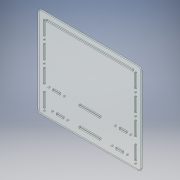
# Autodesk Inventor part: Tapa_Frontal
Saved by Autodesk Inventor 2019 (Build 230136000, 136)
## iProperties
Created: 2020-04-07
Part Number: Tapa_Frontal
Material: Generic
Document SubType Name: Modeling
Designer: Jurgen
Density: 1 g/cm^3
Appearance: Clear
Author: Jurgen
Autodesk Inventor part; units mm, degrees
ref_plane "YZ Plane" through (0, 0, 0) normal (1, 0, 0) x (0, 1, 0)
ref_plane "XZ Plane" through (0, 0, 0) normal (0, 1, 0) x (-1, 0, 0)
ref_plane "XY Plane" through (0, 0, 0) normal (0, 0, 1) x (1, 0, 0)
sketch "Sketch1" plane through (0, 0, 0) normal (0, 0, 1) x (1, 0, 0)
  line L0 (0, 0) -> (20, 0)
  line L1 (0, 0) -> (0, -5)
  line L2 (20, -5) -> (0, -5)
  line L3 (20, 0) -> (20, -5)
  line L4 (76, 0) -> (76, -5)
  line L5 (76, 0) -> (136, 0)
  line L6 (136, -5) -> (76, -5)
  line L7 (136, 0) -> (136, -5)
  line L8 (192, 0) -> (192, -5)
  line L9 (212, 0) -> (192, 0)
  line L10 (212, -5) -> (192, -5)
  line L11 (212, 0) -> (212, -5)
  line L12 (10, -55) -> (10, -60)
  line L13 (30, -55) -> (10, -55)
  line L14 (30, -60) -> (10, -60)
  line L15 (30, -55) -> (30, -60)
  line L16 (76, -55) -> (76, -60)
  line L17 (76, -55) -> (136, -55)
  line L18 (136, -60) -> (76, -60)
  line L19 (136, -55) -> (136, -60)
  line L20 (182, -55) -> (182, -60)
  line L21 (182, -55) -> (202, -55)
  line L22 (202, -60) -> (182, -60)
  line L23 (202, -55) -> (202, -60)
  line L24 (236, -70.0001) -> (236, -80.0001) construction
  line L25 (239.5, -70.0001) -> (236, -70.0001) construction
  line L26 (239.5, -70.0001) -> (239.5, -80.0001) construction
  line L27 (236, -80.0001) -> (239.5, -80.0001) construction
  line L28 (-27.5, -80) -> (-27.5, -70) construction
  line L29 (-24, -70) -> (-27.5, -70) construction
  line L30 (-24, -70) -> (-24, -80) construction
  line L31 (-24, -80) -> (-27.5, -80) construction
  line L32 (-27.5, -60) -> (-27.5, -20)
  line L33 (-24, -20) -> (-27.5, -20)
  line L34 (-24, -60) -> (-24, -20)
  line L35 (-24, -60) -> (-27.5, -60)
  line L36 (-27.5, 0) -> (-27.5, 40)
  line L37 (-24, 40) -> (-24, 0)
  line L38 (-24, 40) -> (-27.5, 40)
  line L39 (-24, 0) -> (-27.5, 0)
  line L40 (-27.5, 60) -> (-27.5, 100)
  line L41 (-24, 100) -> (-27.5, 100)
  line L42 (-24, 100) -> (-24, 60)
  line L43 (-24, 60) -> (-27.5, 60)
  line L44 (-27.5, 160) -> (-27.5, 120)
  line L45 (-24, 160) -> (-24, 120)
  line L46 (-24, 160) -> (-27.5, 160)
  line L47 (236, -0.0001) -> (236, 39.9999)
  line L48 (239.5, 39.9999) -> (239.5, -0.0001)
  line L49 (239.5, 39.9999) -> (236, 39.9999)
  line L50 (239.5, -0.0001) -> (236, -0.0001)
  line L51 (236, -60.0001) -> (236, -20.0001)
  line L52 (239.5, -60.0001) -> (239.5, -20.0001)
  line L53 (239.5, -20.0001) -> (236, -20.0001)
  line L54 (239.5, -60.0001) -> (236, -60.0001)
  line L55 (239.5, 99.9999) -> (236, 99.9999)
  line L56 (236, 59.9999) -> (236, 99.9999)
  line L57 (239.5, 99.9999) -> (239.5, 59.9999)
  line L58 (239.5, 59.9999) -> (236, 59.9999)
  line L59 (236, 159.9999) -> (236, 119.9999)
  line L60 (239.5, 159.9999) -> (239.5, 119.9999)
  line L61 (236, 159.9999) -> (239.5, 159.9999)
  line L62 (236, 111.9999) -> (239.5, 111.9999) construction
  line L63 (239.5, 107.9999) -> (236, 107.9999) construction
  line L64 (236, 51.9999) -> (239.5, 51.9999) construction
  line L65 (239.5, 47.9999) -> (236, 47.9999) construction
  line L66 (236, -66.0001) -> (239.5, -66.0001) construction
  line L67 (212, -60) -> (212, -55) construction
  line L68 (216, -55) -> (216, -60) construction
  line L69 (168, -60) -> (168, -55) construction
  line L70 (172, -55) -> (172, -60) construction
  line L71 (40, -60) -> (40, -55) construction
  line L72 (44, -55) -> (44, -60) construction
  line L73 (-4, -60) -> (-4, -55) construction
  line L74 (0, -55) -> (0, -60) construction
  line L75 (-14, -5) -> (-14, 0) construction
  line L76 (-10, 0) -> (-10, -5) construction
  line L77 (30, -5) -> (30, 0) construction
  line L78 (34, 0) -> (34, -5) construction
  line L79 (178, -5) -> (178, 0) construction
  line L80 (182, 0) -> (182, -5) construction
  line L81 (222, -5) -> (222, 0) construction
  line L82 (226, 0) -> (226, -5) construction
  line L83 (-27.5, -66) -> (-24, -66) construction
  line L84 (-27.5, 52) -> (-24, 52) construction
  line L85 (-24, 48) -> (-27.5, 48) construction
  line L86 (-24, 108) -> (-27.5, 108) construction
  line L87 (-27.5, 112) -> (-24, 112) construction
  line L88 (-24, 120) -> (-27.5, 120)
  line L89 (239.5, 119.9999) -> (236, 119.9999)
  line L90 (-25.75, 112) -> (-25.75, 108) construction
  circle A0 centre (-25.75, 110) radius 2
  line L91 (-25.75, 52) -> (-25.75, 48) construction
  circle A1 centre (-25.75, 50) radius 2
  line L92 (-25.75, -66) -> (-25.75, -70) construction
  circle A2 centre (-25.75, -68) radius 2
  line L93 (237.75, 111.9999) -> (237.75, 107.9999) construction
  circle A3 centre (237.75, 109.9999) radius 2
  line L94 (237.75, 51.9999) -> (237.75, 47.9999) construction
  circle A4 centre (237.75, 49.9999) radius 2
  line L95 (237.75, -66.0001) -> (237.75, -70.0001) construction
  circle A5 centre (237.75, -68.0001) radius 2
  line L96 (-14, -2.5) -> (-10, -2.5) construction
  line L97 (30, -2.5) -> (34, -2.5) construction
  line L98 (178, -2.5) -> (182, -2.5) construction
  line L99 (222, -2.5) -> (226, -2.5) construction
  line L100 (212, -57.5) -> (216, -57.5) construction
  line L101 (168, -57.5) -> (172, -57.5) construction
  line L102 (40, -57.5) -> (44, -57.5) construction
  line L103 (-4, -57.5) -> (0, -57.5) construction
  circle A6 centre (-12, -2.5) radius 2
  circle A7 centre (32, -2.5) radius 2
  circle A8 centre (180, -2.5) radius 2
  circle A9 centre (224, -2.5) radius 2
  circle A10 centre (214, -57.5) radius 2
  circle A11 centre (170, -57.5) radius 2
  circle A12 centre (42, -57.5) radius 2
  circle A13 centre (-2, -57.5) radius 2
  line L104 (-27.5, -80) -> (-42.5, -80) construction
  line L105 (239.5, 159.9999) -> (254.5, 159.9999) construction
  line L106 (254.5, 159.9999) -> (254.5, 179.9999) construction
  line L107 (254.5, 179.9999) -> (239.5, 179.9999) construction
  line L108 (239.5, 179.9999) -> (239.5, 159.9999) construction
  line L109 (254.5, 179.9999) -> (-42.5, 179.9999)
  line L110 (-42.5, 179.9999) -> (-42.5, -80)
  line L111 (-42.5, -80) -> (254.5, -80)
  line L112 (254.5, -80) -> (254.5, 179.9999)
  dimension "d0" = 15
  dimension "d3" = 15
  dimension "d4" = 20
  constraints: 226 end point, 42 midpoint, 8 horizontal alignment, 6 vertical alignment, 4 parallel, 3 horizontal, 2 perpendicular, 28 other
  measures "d0" distance of L28.start L104.end
  measures "d3" distance of L107.end L106.end
  measures "d4" distance of L106.end L105.end
extrude "Extrusion1" add sketch "Sketch1" along normal blind 3.5
fillet "Fillet1" radius 8 4 edges at (254.5, 179.9999, 1.75) (-42.5, 179.9999, 1.75) (254.5, -80, 1.75) (-42.5, -80, 1.75)
sketch "Sketch2" plane through (0, 0, 3.5) normal (0, 0, 1) x (1, 0, 0)
  arc A0 (-42.5, -72) -> (-34.5, -80) centre (-34.5, -72) ccw construction
  line L0 (-34.5, -80) -> (246.5, -80) construction
  arc A1 (246.5, -80) -> (254.5, -72) centre (246.5, -72) ccw construction
  line L1 (254.5, -72) -> (254.5, 171.9999) construction
  arc A2 (254.5, 171.9999) -> (246.5, 179.9999) centre (246.5, 171.9999) ccw construction
  line L2 (246.5, 179.9999) -> (-34.5, 179.9999) construction
  arc A3 (-34.5, 179.9999) -> (-42.5, 171.9999) centre (-34.5, 171.9999) ccw construction
  line L3 (-42.5, 171.9999) -> (-42.5, -72) construction
  line L4 (76, -55) -> (136, -55) construction
  line L5 (136, -55) -> (136, -60) construction
  line L6 (136, -60) -> (76, -60) construction
  line L7 (76, -60) -> (76, -55) construction
  line L8 (76, 0) -> (136, 0) construction
  line L9 (136, 0) -> (136, -5) construction
  line L10 (136, -5) -> (76, -5) construction
  line L11 (76, -5) -> (76, 0) construction
  line L12 (236, 159.9999) -> (239.5, 159.9999) construction
  line L13 (239.5, 159.9999) -> (239.5, 119.9999) construction
  line L14 (239.5, 119.9999) -> (236, 119.9999) construction
  line L15 (236, 119.9999) -> (236, 159.9999) construction
  line L16 (239.5, 99.9999) -> (239.5, 59.9999) construction
  line L17 (239.5, 59.9999) -> (236, 59.9999) construction
  line L18 (236, 59.9999) -> (236, 99.9999) construction
  line L19 (236, 99.9999) -> (239.5, 99.9999) construction
  line L20 (236, -20.0001) -> (239.5, -20.0001) construction
  line L21 (239.5, -20.0001) -> (239.5, -60.0001) construction
  line L22 (239.5, -60.0001) -> (236, -60.0001) construction
  line L23 (236, -60.0001) -> (236, -20.0001) construction
  line L24 (236, 39.9999) -> (239.5, 39.9999) construction
  line L25 (239.5, 39.9999) -> (239.5, -0.0001) construction
  line L26 (239.5, -0.0001) -> (236, -0.0001) construction
  line L27 (236, -0.0001) -> (236, 39.9999) construction
  line L28 (-27.5, 160) -> (-24, 160) construction
  line L29 (-24, 160) -> (-24, 120) construction
  line L30 (-24, 120) -> (-27.5, 120) construction
  line L31 (-27.5, 120) -> (-27.5, 160) construction
  line L32 (-27.5, 100) -> (-24, 100) construction
  line L33 (-24, 100) -> (-24, 60) construction
  line L34 (-24, 60) -> (-27.5, 60) construction
  line L35 (-27.5, 60) -> (-27.5, 100) construction
  line L36 (-27.5, 40) -> (-24, 40) construction
  line L37 (-24, 40) -> (-24, 0) construction
  line L38 (-24, 0) -> (-27.5, 0) construction
  line L39 (-27.5, 0) -> (-27.5, 40) construction
  line L40 (-27.5, -20) -> (-24, -20) construction
  line L41 (-24, -20) -> (-24, -60) construction
  line L42 (-24, -60) -> (-27.5, -60) construction
  line L43 (-27.5, -60) -> (-27.5, -20) construction
  line L44 (182, -55) -> (202, -55) construction
  line L45 (202, -55) -> (202, -60) construction
  line L46 (202, -60) -> (182, -60) construction
  line L47 (182, -60) -> (182, -55) construction
  line L48 (10, -55) -> (30, -55) construction
  line L49 (30, -55) -> (30, -60) construction
  line L50 (30, -60) -> (10, -60) construction
  line L51 (10, -60) -> (10, -55) construction
  line L52 (192, 0) -> (212, 0) construction
  line L53 (212, 0) -> (212, -5) construction
  line L54 (212, -5) -> (192, -5) construction
  line L55 (192, -5) -> (192, 0) construction
  line L56 (20, 0) -> (20, -5) construction
  line L57 (20, -5) -> (0, -5) construction
  line L58 (0, -5) -> (0, 0) construction
  line L59 (0, 0) -> (20, 0) construction
  circle A4 centre (-2, -57.5) radius 2 construction
  circle A5 centre (42, -57.5) radius 2 construction
  circle A6 centre (170, -57.5) radius 2 construction
  circle A7 centre (214, -57.5) radius 2 construction
  circle A8 centre (224, -2.5) radius 2 construction
  circle A9 centre (180, -2.5) radius 2 construction
  circle A10 centre (32, -2.5) radius 2 construction
  circle A11 centre (-12, -2.5) radius 2 construction
  circle A12 centre (237.75, -68.0001) radius 2 construction
  circle A13 centre (237.75, 49.9999) radius 2 construction
  circle A14 centre (237.75, 109.9999) radius 2 construction
  circle A15 centre (-25.75, -68) radius 2 construction
  circle A16 centre (-25.75, 50) radius 2 construction
  circle A17 centre (-25.75, 110) radius 2 construction
  line L60 (-24, 160) -> (236, 159.9999) construction
  line L61 (-19, 160) -> (231, 160)
  line L62 (231, 160) -> (231, 163.5)
  line L63 (231, 163.5) -> (-19, 163.5)
  line L64 (-19, 163.5) -> (-19, 160)
  dimension "d8" = 250
  dimension "d9" = 3.5
  dimension "d10" = 5
  constraints: 10 end point, 2 parallel, 1 horizontal, 1 perpendicular, 1 point on line
  measures "d8" distance of L63.end L62.end
  measures "d9" distance of L61.end L62.end
  measures "d10" distance between parallel lines of L29 L64
extrude "Extrusion2" cut sketch "Sketch2" against normal blind 3.5
body "Solid1"
